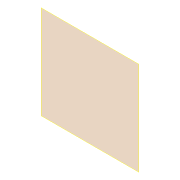
# Autodesk Inventor part: 01_bridge_raspberrypicam_zfocus
Saved by Autodesk Inventor 2019.4 (Build 234330000, 330)
## iProperties
Created: 2020-10-20
Part Number: 01_bridge_raspberrypicam_zfocus
Material: Generic
Document SubType Name: Modeling
Designer: diederichbenedict
Density: 1 g/cm^3
Appearance: Default
Author: diederichbenedict
Autodesk Inventor part; units mm, degrees
ref_plane "YZ Plane" through (0, 0, 0) normal (1, 0, 0) x (0, 1, 0)
ref_plane "XZ Plane" through (0, 0, 0) normal (0, 1, 0) x (-1, 0, 0)
ref_plane "XY Plane" through (0, 0, 0) normal (0, 0, 1) x (1, 0, 0)
ref_plane "Work Plane2" through (-7.6233, -13.6279, 6) normal (0, 0, 1) x (0.9998, 0.0187, 0)
sketch "Sketch1" plane through (-7.6233, -13.6279, 6) normal (0, 0, 1) x (0.9998, 0.0187, 0)
  arc A0 (8.7735, -0.0173) -> (8.7735, 0.8133) centre (8.2735, 0.398) ccw construction
  line L0 (8.7735, -0.0173) -> (8.7735, -8.102) construction
  line L1 (8.7735, -8.102) -> (1.4505, -8.102) construction
  arc A1 (-1.9036, -8.102) -> (1.4505, -8.102) centre (-0.2265, -8.602) ccw construction
  line L2 (-1.9036, -8.102) -> (-8.2265, -8.102) construction
  line L3 (-8.2265, -8.102) -> (-8.2265, -4.0381) construction
  arc A2 (-8.2265, -1.1658) -> (-8.2265, -4.0381) centre (-9.2265, -2.602) ccw construction
  line L4 (-8.2265, -1.1658) -> (-8.2265, 7.898) construction
  line L5 (-8.2265, 7.898) -> (-1.7274, 7.898) construction
  arc A3 (1.2743, 7.898) -> (-1.7274, 7.898) centre (-0.2265, 8.798) ccw construction
  line L6 (1.2743, 7.898) -> (8.7735, 7.898) construction
  line L7 (8.7735, 7.898) -> (8.7735, 5.6221) construction
  arc A4 (8.7735, 2.1739) -> (8.7735, 5.6221) centre (9.0735, 3.898) ccw construction
  line L8 (8.7735, 2.1739) -> (8.7735, 0.8133) construction
  circle A5 centre (-9.2265, -7.102) radius 0.65 construction
  line L9 (-9.6265, 5.198) -> (-14.4265, 5.198) construction
  line L10 (-14.4265, 5.198) -> (-19.2265, 5.198) projected
  line L11 (-19.2265, 5.198) -> (-19.2265, -11.602) projected
  line L12 (-19.2265, -11.602) -> (11.2735, -11.602) projected
  line L13 (11.2735, -11.602) -> (11.2735, 14.798) construction
  line L14 (11.2735, 14.798) -> (-9.6265, 14.798) construction
  line L15 (-9.6265, 14.798) -> (-9.6265, 9.998) construction
  line L16 (-9.6265, 9.998) -> (-9.6265, 5.198) construction
  arc A6 (8.7735, 0.8133) -> (8.7735, -0.0173) centre (8.2735, 0.398) ccw construction
  line L17 (8.7735, 0.8133) -> (8.7735, 2.1739) construction
  arc A7 (8.7735, 2.1739) -> (8.7735, 5.6221) centre (9.0735, 3.898) ccw construction
  line L18 (8.7735, 5.6221) -> (8.7735, 7.898) construction
  line L19 (8.7735, 7.898) -> (1.2743, 7.898) construction
  arc A8 (1.2743, 7.898) -> (-1.7274, 7.898) centre (-0.2265, 8.798) ccw construction
  line L20 (-1.7274, 7.898) -> (-8.2265, 7.898) construction
  line L21 (-8.2265, 7.898) -> (-8.2265, -1.1658) construction
  arc A9 (-8.2265, -1.1658) -> (-8.2265, -4.0381) centre (-9.2265, -2.602) ccw construction
  line L22 (-8.2265, -4.0381) -> (-8.2265, -8.102) construction
  line L23 (-8.2265, -8.102) -> (-1.9036, -8.102) construction
  arc A10 (-1.9036, -8.102) -> (1.4505, -8.102) centre (-0.2265, -8.602) ccw construction
  line L24 (1.4505, -8.102) -> (8.7735, -8.102) construction
  line L25 (8.7735, -8.102) -> (8.7735, -0.0173) construction
  line L26 (-6.2265, -6.102) -> (-6.2265, 5.898) construction
  line L27 (-6.2265, 5.898) -> (6.7735, 5.898) construction
  line L28 (6.7735, 5.898) -> (6.7735, -6.102) construction
  line L29 (6.7735, -6.102) -> (-6.2265, -6.102) construction
  circle A11 centre (-9.2265, -2.602) radius 0.9 construction
  circle A12 centre (9.0735, 3.898) radius 0.9 construction
  circle A13 centre (-0.2265, 8.798) radius 0.9 construction
  circle A14 centre (-0.2265, -8.602) radius 0.9 construction
  line L30 (10.1735, -9.602) -> (10.1735, -4.102) construction
  line L31 (12.2735, -9.602) -> (10.1735, -9.602) construction
  line L32 (12.2735, 14.398) -> (12.2735, -9.602) construction
  line L33 (-12.7265, 14.398) -> (12.2735, 14.398) construction
  line L34 (-12.7265, -9.602) -> (-12.7265, 14.398) construction
  line L35 (-10.6265, -9.602) -> (-12.7265, -9.602) construction
  line L36 (-10.6265, -4.102) -> (-10.6265, -9.602) construction
  line L37 (10.1735, -4.102) -> (-10.6265, -4.102) construction
  circle A15 centre (10.2735, 12.398) radius 1.05 construction
  circle A16 centre (10.2735, -0.102) radius 1.05 construction
  circle A17 centre (-10.7265, -0.102) radius 1.05 construction
  circle A18 centre (-10.7265, 12.398) radius 1.05 construction
  line L38 (8.7735, 0.798) -> (8.7735, 12.398) construction
  line L39 (-8.9265, 0.798) -> (8.7735, 0.798) construction
  line L40 (-8.9265, 12.398) -> (-8.9265, 0.798) construction
  line L41 (8.7735, 12.398) -> (-8.9265, 12.398) construction
  line L42 (12.2735, 14.398) -> (-12.7265, 14.398)
  line L43 (-12.7265, 14.398) -> (-12.7265, -9.602)
  line L44 (-12.7265, -9.602) -> (12.2735, -9.602)
  line L45 (12.2735, -9.602) -> (12.2735, 14.398)
  circle A19 centre (9.0735, 3.898) radius 1
  circle A20 centre (-0.2265, 8.798) radius 1
  circle A21 centre (-0.2265, -8.602) radius 1
  circle A22 centre (-9.2265, -2.602) radius 1
  circle A23 centre (-0.2265, -0.102) radius 2.8 projected
  circle A24 centre (-0.2265, -0.102) radius 7.5
  point P0 (7.8766, 13.4831)
  dimension "d0" = 2
  dimension "d1" = 2
  dimension "d2" = 2
  dimension "d3" = 2
  dimension "d4" = 15
  constraints: 8 end point, 5 centre point, 5 coincident, 2 parallel, 1 horizontal, 1 perpendicular
  measures "d0" diameter of A19
  measures "d1" diameter of A20
  measures "d2" diameter of A21
  measures "d3" diameter of A22
  measures "d4" diameter of A24
extrude "Extrusion1" add sketch "Sketch1" along normal blind 2 contours L45 L44 L43 L42
sketch "Sketch2" plane through (-7.8479, -13.7341, 8) normal (0, 0, 1) x (1, 0, 0)
  point P0 (7.8479, 13.7341)
body "Solid1"
